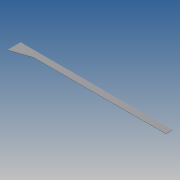
# Autodesk Inventor part: sidewalkBack
Saved by Autodesk Inventor 2013 (Build 170138000, 138)
## iProperties
Created: 2014-01-02
Part Number: sidewalkBack
Material: Generic
Document SubType Name: Modeling
Designer: ddeboer
Density: 1 g/cm^3
Author: ddeboer
Autodesk Inventor part; units mm, degrees
ref_plane "YZ Plane" through (0, 0, 0) normal (1, 0, 0) x (0, 1, 0)
ref_plane "XZ Plane" through (0, 0, 0) normal (0, 1, 0) x (-1, 0, 0)
ref_plane "XY Plane" through (0, 0, 0) normal (0, 0, 1) x (1, 0, 0)
sketch "Sketch1" plane through (0, 0, 0) normal (0, 1, 0) x (-1, 0, 0)
  line L0 (0, 0) -> (1524, 0)
  line L1 (1524, 0) -> (1524, 1016)
  line L2 (1524, 1016) -> (0, 508)
  line L3 (0, 0) -> (-10363.2, 0)
  line L4 (0, 508) -> (-10363.2, 508)
  line L5 (-10363.2, 508) -> (-10363.2, 0)
  dimension "d0" = 1524
  dimension "d1" = 508
  dimension "d2" = 1016
  dimension "d3" = 10363.2
  dimension "d4" = 10363.2
  constraints: 12 end point, 2 perpendicular, 1 horizontal, 1 parallel
  measures "d0" distance of L0.start L0.end
  measures "d1" distance of L0.start L2.end
  measures "d2" distance of L0.end L1.end
  measures "d3" distance of L0.start L3.end
  measures "d4" distance of L2.end L4.end
extrude "Extrusion1" add sketch "Sketch1" along normal blind 25.4
body "Solid1"
